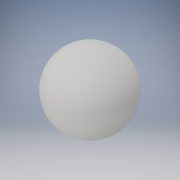
# Autodesk Inventor part: dracothruster
Saved by Autodesk Inventor 2018 (Build 220112000, 112)
## iProperties
Created: 2018-04-22
Part Number: dracothruster
Material: Generic
Document SubType Name: Modeling
Designer: atbin
Density: 0.231958 g/cm^3
Appearance: Default
Mass: 15181.6 g
Surface Area: 7853.98 cm^2
Volume: 65449.8 cm^3
Author: atbin
Autodesk Inventor part; units mm, degrees
ref_plane "YZ Plane" through (0, 0, 0) normal (1, 0, 0) x (0, 1, 0)
ref_plane "XZ Plane" through (0, 0, 0) normal (0, 1, 0) x (-1, 0, 0)
ref_plane "XY Plane" through (0, 0, 0) normal (0, 0, 1) x (1, 0, 0)
sketch "Sketch1" plane through (0, 0, 0) normal (0, 0, 1) x (1, 0, 0)
  arc A0 (0, -250) -> (0, 250) centre (0, 0) ccw
  line L0 (0, 250) -> (0, -250)
  dimension "d0" = 500
  dimension "d1" = 0
  constraints: 2 end point, 2 point on circle, 1 centre point, 1 vertical
  measures "d0" diameter of A0
  measures "d1" distance of point (0, 0) A0.centre
revolve "Revolution1" add sketch "Sketch1" angle 360 about axis through (0, 250, 0) along (0, -1, 0)
body "Solid1"
